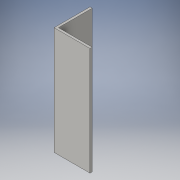
# Autodesk Inventor part: gripper limiter brackets
Saved by Autodesk Inventor 2016 SP2 (Build 200236200, 236)
## iProperties
Created: 2018-02-13
Part Number: gripper limiter brackets
Material: Generic
Document SubType Name: Modeling
Designer: CAD
Density: 1 g/cm^3
Appearance: Default
Author: CAD
Autodesk Inventor part; units mm, degrees
ref_plane "YZ Plane" through (0, 0, 0) normal (1, 0, 0) x (0, 1, 0)
ref_plane "XZ Plane" through (0, 0, 0) normal (0, 1, 0) x (-1, 0, 0)
ref_plane "XY Plane" through (0, 0, 0) normal (0, 0, 1) x (1, 0, 0)
sketch "Sketch1" plane through (0, 0, 0) normal (0, 1, 0) x (-1, 0, 0)
  line L0 (0, 0) -> (0, -25.4)
  line L1 (0, 0) -> (-25.4, 0)
  line L2 (-1.5875, -25.4) -> (-1.5875, -1.5875)
  line L3 (-1.5875, -1.5875) -> (-25.4, -1.5875)
  line L4 (0, -25.4) -> (-1.5875, -25.4)
  line L5 (-25.4, 0) -> (-25.4, -1.5875)
  point P0 (0, -12.7)
  dimension "d1" = 25.4
  dimension "d2" = 25.4
  dimension "d3" = 1.5875
  constraints: 12 end point, 2 horizontal, 1 midpoint, 1 perpendicular, 1 vertical, 1 other
  measures "d1" distance of L0.start L1.end
  measures "d2" distance of L0.start L0.end
  measures "d3" distance between parallel lines of L0 L2
extrude "Extrusion1" add sketch "Sketch1" along normal blind 76.2
body "Solid1"
